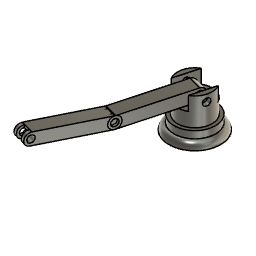
Mani v6 (Autodesk Fusion 360 design; units mm, degrees)
Autodesk Fusion 360 part; units mm, degrees
sketch "Sketch1" plane through (0, 0, 0) normal (0, 0, 1) x (1, 0, 0)
  circle A0 centre (0, 0) radius 25
  dimension "d1" = 50
  constraint coincident A0.centre origin
  measures "d1" diameter of A0
extrude "Extrude1" add sketch "Sketch1" along normal blind 10 makes body 1
sketch "Sketch2" plane through (0, 0, 10) normal (0, 0, 1) x (-1, 0, 0)
  circle A0 centre (0, 0) radius 25
  circle A1 centre (0, 0) radius 5
  dimension "d4" = 10
  constraint concentric A0 A1
  measures "d4" diameter of A1
extrude "Extrude2" add sketch "Sketch2" along normal blind 20 contours A1 bodies 1
sketch "Sketch5" plane through (0, 0, 10) normal (0, 0, 1) x (-1, 0, 0)
  circle A0 centre (0, 0) radius 5
  circle A1 centre (0, 0) radius 25
  circle A2 centre (0, 0) radius 25
  constraint coincident A0.centre A1.centre
extrude "Extrude1'" add sketch "Sketch5" along normal blind 20 separate body makes body 2 in component "Component"
sketch "Sketch6" plane through (0, 0, 30) normal (0, 0, 1) x (-1, 0, 0)
  circle A0 centre (0, 0) radius 5
  circle A1 centre (0, 0) radius 25
  line L0 (17.6777, 17.6777) -> (17.6777, -17.6777)
  line L1 (-17.6777, -17.6777) -> (-17.6777, 17.6777)
  line L2 (-17.6777, 17.6777) -> (17.6777, -17.6777) construction
  line L3 (17.6777, 17.6777) -> (-17.6777, -17.6777) construction
  arc A2 (17.6777, -17.6777) -> (17.6777, 17.6777) centre (0, 0) ccw
  arc A3 (-17.6777, 17.6777) -> (-17.6777, -17.6777) centre (0, 0) ccw
  dimension "d20" = 50
  dimension "d22" = 35.3553
  dimension "d23" = 35.3553
  constraint concentric A0 A2
  constraint parallel L0 L1
  constraint coincident L1.end A2
  constraint coincident L2 A0.centre
  constraint coincident L3 A0.centre
  constraint coincident A0.centre A1.centre
  constraint concentric A2 A3
  measures "d20" diameter of A2
  measures "d22" distance of L0.end L1.start
  measures "d23" distance of L0.start L0.end
extrude "Extrude2'" add sketch "Sketch6" along normal blind 20 contours A1 L0 A2 | A1 L1 A3 bodies 2 in component "Component"
sketch "Sketch7" plane through (-17.6777, 0, 0) normal (1, 0, 0) x (0, 1, 0)
  line L0 (-17.6777, 30) -> (17.6777, 30)
  line L1 (17.6777, 30) -> (17.6777, 50)
  line L2 (17.6777, 50) -> (-17.6777, 50)
  line L3 (-17.6777, 50) -> (-17.6777, 30)
  circle A0 centre (0, 40) radius 5
  line L4 (25, 30) -> (17.6777, 30)
  dimension "d26" = 10
  dimension "d46" = 10
  dimension "d47" = 20
  measures "d26" diameter of A0
  measures "d46" distance of A0.centre L4
  measures "d47" distance of L0 L2
extrude "Extrude3" cut sketch "Sketch7" along normal blind 50 and the other way blind 35 contours A0 bodies 2 in component "Component"
extrude "Extrude1''" add sketch "Sketch7" along normal blind 30 and the other way blind 0 separate body contours A0 makes body 3 in component "Component'"
sketch "Sketch8" plane through (0, 0, 0) normal (1, 0, 0) x (0, 1, 0)
  circle A0 centre (0, 40) radius 5
  line L0 (0, 48.5) -> (-100, 48.5)
  arc A1 (-100, 48.5) -> (-100, 31.5) centre (-100, 40) ccw
  line L1 (-100, 31.5) -> (0, 31.5)
  arc A2 (0, 31.5) -> (0, 48.5) centre (0, 40) ccw
  line L2 (0, 40) -> (-100, 40) construction
  circle A3 centre (-100, 40) radius 5
  point P0 (0, 40)
  dimension "d48" = 10
  dimension "d49" = 17
  dimension "d51" = 100
  dimension "d56" = 10
  constraint tangent L0 A1
  constraint tangent A1 L1
  constraint parallel L0 L1
  constraint tangent L1 A2
  constraint tangent L0 A2
  constraint horizontal L2
  constraint coincident P0 A0.centre
  constraint concentric A1 A3
  measures "d48" diameter of A0
  measures "d49" diameter of A1
  measures "d51" distance of A1.end L1.end
  measures "d56" diameter of A3
extrude "Extrude2''" add sketch "Sketch8" along normal blind 10 and the other way blind 10 sketch seen with x (1, 0, 0) y (0, 1, 0) z (0, 0, 1) at (-9.0177, 0, 0) bodies 3 in component "Component'"
sketch "Sketch9" plane through (0, 0, 0) normal (0, 0, -1) x (1, 0, 0)
  circle A0 centre (0, 0) radius 25
  circle A1 centre (0, 0) radius 37.5
  dimension "d61" = 75
  constraint concentric A0 A1
  measures "d61" diameter of A1
extrude "Extrude3'" add sketch "Sketch9" along normal blind 10 contours A0 | A1 bodies 1
fillet "Fillet1" radius 10 1 edges at (-34.9623, 13.5606, 0) on bodies 1
move_face "OffsetFaces1" offset 5 1 faces at (-24.9689, 1.2461, 3.3333) on bodies 1
sketch "Sketch10" plane through (21.3401, 0, 0) normal (1, 0, 0) x (0, 1, 0)
  circle A0 centre (-100, 40) radius 5
  circle A1 centre (-100, 40) radius 5
  dimension "d67" = 10
  constraint concentric A0 A1
  measures "d67" diameter of A1
extrude "Extrude3''" cut sketch "Sketch10" against normal blind 15 sketch seen with x (1, 0, 0) y (0, 1, 0) z (0, 0, 1) at (-9.0177, 100, 0) bodies 3 in component "Component'"
sketch "Sketch11" plane through (0, 0, 48.5) normal (0, 0, 1) x (-1, 0, 0)
  line L0 (10, 200) -> (-10, 200)
  line L1 (-10, 200) -> (-10, 100)
  line L2 (-10, 100) -> (10, 100)
  line L3 (10, 100) -> (10, 200)
  line L4 (-5, 200) -> (5, 200)
  line L5 (5, 200) -> (5, 280)
  line L6 (5, 280) -> (-5, 280)
  line L7 (-5, 280) -> (-5, 200)
  line L8 (-5, 200) -> (5, 280) construction
  line L9 (5, 200) -> (-5, 280) construction
  point P0 (0, 240)
  dimension "d70" = 10
  constraint horizontal L4
  constraint perpendicular L4 L5
  constraint parallel L4 L6
  constraint parallel L5 L7
  constraint coincident L8 P0
  constraint coincident L9 P0
  measures "d70" distance of L5.end L6.end
extrude "Extrude4" cut sketch "Sketch11" against normal blind 40 contours L0 L4 L5 L6 L7 sketch seen with x (1, 0, 0) y (0, 1, 0) z (0, 0, 1) at (-9.0177, 100, 0) bodies 3 in component "Component'"
component "Component" placed x (1, 0, 0) y (0, 1, 0) z (0, 0, 1) at (0, 0, 0)
component "Component'" placed x (1, 0, 0) y (0, 1, 0) z (0, 0, 1) at (9.0177, 0, 0)
component "Component'" placed x (1, 0, 0) y (0, 1, 0) z (0, 0, 1) at (9.0177, -100, 0)
